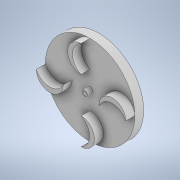
# Autodesk Inventor part: 20220701_fan_wing4
Saved by Autodesk Inventor 2020 (Build 240168000, 168)
## iProperties
Created: 2022-06-29
Part Number: 20220701_fan_wing4
Material: 一般
Document SubType Name: Modeling
Designer: Naggy
Density: 1 g/cm^3
Appearance: 既定
Author: Naggy
Autodesk Inventor part; units mm, degrees
ref_plane "YZ Plane" through (0, 0, 0) normal (1, 0, 0) x (0, 1, 0)
ref_plane "XZ Plane" through (0, 0, 0) normal (0, 1, 0) x (-1, 0, 0)
ref_plane "XY Plane" through (0, 0, 0) normal (0, 0, 1) x (1, 0, 0)
sketch "スケッチ1" plane through (0, 0, 0) normal (0, 0, 1) x (1, 0, 0)
  circle A0 centre (0, 0) radius 25
  dimension "d0" = 50
  constraints: 1 centre point, 1 coincident
  measures "d0" diameter of A0
extrude "押し出し1" add sketch "スケッチ1" along normal blind 5
sketch "スケッチ2" plane through (0, 0, 5) normal (0, 0, 1) x (1, 0, 0)
  circle A0 centre (0, 0) radius 10
  circle A1 centre (0, 0) radius 25 projected
  arc A2 (0, 25) -> (0, 10) centre (0, 17.5) ccw
  arc A3 (0, 25) -> (0, 10) centre (3.5, 17.5) ccw
  arc A4 (-25, 0) -> (-10, 0) centre (-17.5, 3.5) ccw
  arc A5 (-25, 0) -> (-10, 0) centre (-17.5, 0) ccw
  arc A6 (0, -25) -> (0, -10) centre (-3.5, -17.5) ccw
  arc A7 (0, -25) -> (0, -10) centre (0, -17.5) ccw
  arc A8 (25, 0) -> (10, 0) centre (17.5, -3.5) ccw
  arc A9 (25, 0) -> (10, 0) centre (17.5, 0) ccw
  dimension "d3" = 20
  dimension "d4" = 3.5
  dimension "d7" = 360
  constraints: 16 point on circle, 8 centre point, 2 vertical alignment, 1 coincident, 29 other
  measures "d4" distance of A3.centre A2.centre
extrude "押し出し2" add sketch "スケッチ2" along normal blind 5 contours A9 A8 | A2 A3 | A7 A6 | A5 A4
sketch "スケッチ3" plane through (0, 0, 5) normal (0, 0, 1) x (1, 0, 0)
  point P0 (0, 0)
  point P1 (0, 0)
  constraints: 1 coincident
hole "穴1" at (0, 0, 5) direction (0, 0, -1) diameter 1.9 depth 6 tip angle 118
sketch "スケッチ4" plane through (0, 0, 5) normal (0, 0, 1) x (1, 0, 0)
  circle A0 centre (0, 0) radius 0.95 projected
  circle A1 centre (0, 0) radius 1.5
  dimension "d18" = 3
  constraints: 1 centre point, 1 coincident
  measures "d18" diameter of A1
extrude "押し出し3" add sketch "スケッチ4" along normal blind 3
sketch "スケッチ5" plane through (0, 0, 0) normal (1, 0, 0) x (0, 1, 0)
  line L0 (0, 5) -> (0, 10) projected
  point P0 (0, 0)
  point P1 (0, 6.3224)
  constraints: 1 point on line
hole "穴2" at (0, 0, 6.3224) direction (-1, 0, 0) diameter 1 depth 2 tip angle 118
